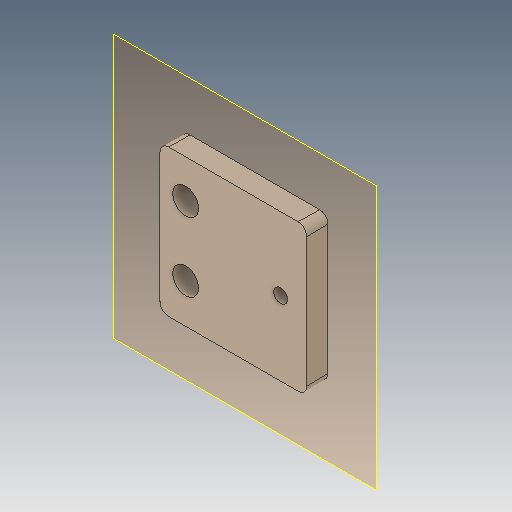
# Autodesk Inventor part: 30_Cube_Z_Focus_Drylin_NEMA_counterplate
Saved by Autodesk Inventor 2019.4 (Build 234330000, 330)
## iProperties
Created: 2021-05-03
Part Number: 30_Cube_Z_Focus_Drylin_NEMA_counterplate
Material: Generic
Document SubType Name: Modeling
Designer: diederichbenedict
Density: 1 g/cm^3
Appearance: Default
Author: diederichbenedict
Autodesk Inventor part; units mm, degrees
ref_plane "YZ Plane" through (0, 0, 0) normal (1, 0, 0) x (0, 1, 0)
ref_plane "XZ Plane" through (0, 0, 0) normal (0, 1, 0) x (-1, 0, 0)
ref_plane "XY Plane" through (0, 0, 0) normal (0, 0, 1) x (1, 0, 0)
ref_plane "Work Plane1" through (15.4052, 15.0652, 4.9) normal (0, 0, 1) x (0, 1, 0)
sketch "Sketch1" plane through (15.4052, 15.0652, 4.9) normal (0, 0, 1) x (0, 1, 0)
  circle A0 centre (5.7948, 15.4052) radius 2.5 projected
  circle A1 centre (-15.6052, -5.7948) radius 2.5 projected
  line L0 (-20.0856, 39.0762) -> (-20.0856, 40.2052) projected
  line L1 (-20.0856, 40.2052) -> (-38.2052, 40.2052) projected
  arc A2 (-38.2052, 40.2052) -> (-40.2052, 38.2052) centre (-38.2052, 38.2052) ccw projected
  line L2 (-40.2052, 20.2953) -> (-40.2052, 38.2052) projected
  line L3 (-40.2052, 20.2953) -> (-39.0783, 20.2953) projected
  arc A3 (-39.0783, 20.2953) -> (-38.6768, 20.6232) centre (-39.0783, 20.7051) ccw projected
  arc A4 (-34.5391, 20.2052) -> (-38.6768, 20.6232) centre (-36.6291, 20.2052) ccw projected
  line L4 (-34.5391, 20.2052) -> (-34.5391, 10.4067) projected
  arc A5 (-38.647, 9.8643) -> (-34.5391, 10.4067) centre (-36.6023, 10.2052) ccw projected
  line L5 (-38.647, 9.8643) -> (-38.6775, 9.9849) projected
  arc A6 (-38.6775, 9.9849) -> (-39.0762, 10.3249) centre (-39.083, 9.9131) ccw projected
  line L6 (-39.0762, 10.3249) -> (-40.2052, 10.3249) projected
  line L7 (-40.2052, -7.7948) -> (-40.2052, 10.3249) projected
  arc A7 (-40.2052, -7.7948) -> (-38.2052, -9.7948) centre (-38.2052, -7.7948) ccw projected
  line L8 (-38.2052, -9.7948) -> (-20.2052, -9.7948) projected
  line L9 (-20.2052, -9.7948) -> (-20.2052, -10.8453) projected
  arc A8 (-20.6052, -11.3352) -> (-20.2052, -10.8453) centre (-20.7052, -10.8453) ccw projected
  arc A9 (-20.6052, -11.3352) -> (-20.2052, -15.2948) centre (-20.2052, -13.2948) ccw projected
  line L10 (-20.2052, -15.2948) -> (-10.2052, -15.2948) projected
  arc A10 (-10.2052, -15.2948) -> (-9.8052, -11.3352) centre (-10.2052, -13.2948) ccw projected
  arc A11 (-10.2052, -10.8453) -> (-9.8052, -11.3352) centre (-9.7052, -10.8453) ccw projected
  line L11 (-10.2052, -10.8453) -> (-10.2052, -9.7948) projected
  line L12 (-10.2052, -9.7948) -> (7.7948, -9.7948) projected
  arc A12 (7.7948, -9.7948) -> (9.7948, -7.7948) centre (7.7948, -7.7948) ccw projected
  line L13 (9.7948, 10.2052) -> (9.7948, -7.7948) projected
  line L14 (9.7948, 10.2052) -> (10.8453, 10.2052) projected
  arc A13 (11.3352, 9.8052) -> (10.8453, 10.2052) centre (10.8453, 9.7052) ccw projected
  arc A14 (11.3352, 9.8052) -> (15.2948, 10.2052) centre (13.2948, 10.2052) ccw projected
  line L15 (15.2948, 10.2052) -> (15.2948, 20.2052) projected
  arc A15 (15.2948, 20.2052) -> (11.3352, 20.6052) centre (13.2948, 20.2052) ccw projected
  arc A16 (10.8453, 20.2052) -> (11.3352, 20.6052) centre (10.8453, 20.7052) ccw projected
  line L16 (10.8453, 20.2052) -> (9.7948, 20.2052) projected
  line L17 (9.7948, 38.2052) -> (9.7948, 20.2052) projected
  arc A17 (9.7948, 38.2052) -> (7.7948, 40.2052) centre (7.7948, 38.2052) ccw projected
  line L18 (7.7948, 40.2052) -> (-10.1151, 40.2052) projected
  line L19 (-10.1151, 40.2052) -> (-10.1151, 39.0783) projected
  arc A18 (-10.1151, 39.0783) -> (-9.7873, 38.6768) centre (-9.7054, 39.0783) ccw projected
  arc A19 (-10.2052, 34.5391) -> (-9.7873, 38.6768) centre (-10.2052, 36.6291) ccw projected
  line L20 (-10.2052, 34.5391) -> (-20.0038, 34.5391) projected
  arc A20 (-20.5462, 38.647) -> (-20.0038, 34.5391) centre (-20.2052, 36.6023) ccw projected
  line L21 (-20.5462, 38.647) -> (-20.4256, 38.6775) projected
  arc A21 (-20.4256, 38.6775) -> (-20.0856, 39.0762) centre (-20.4974, 39.083) ccw projected
  line L22 (-0.2052, 32.2052) -> (-30.2052, 32.2052) projected
  arc A22 (1.7948, 30.2052) -> (-0.2052, 32.2052) centre (-0.2052, 30.2052) ccw projected
  line L23 (1.7948, 30.2052) -> (1.7948, 0.2052) projected
  arc A23 (-0.2052, -1.7948) -> (1.7948, 0.2052) centre (-0.2052, 0.2052) ccw projected
  line L24 (-0.2052, -1.7948) -> (-30.2052, -1.7948) projected
  arc A24 (-32.2052, 0.2052) -> (-30.2052, -1.7948) centre (-30.2052, 0.2052) ccw projected
  line L25 (-32.2052, 0.2052) -> (-32.2052, 30.2052) projected
  arc A25 (-30.2052, 32.2052) -> (-32.2052, 30.2052) centre (-30.2052, 30.2052) ccw projected
  circle A26 centre (-35.2052, 35.2052) radius 2.425 projected
  circle A27 centre (-29.7052, 36.0052) radius 2.65 projected
  circle A28 centre (-36.0052, 29.7052) radius 2.65 projected
  circle A29 centre (-35.2052, -4.7948) radius 2.425 projected
  circle A30 centre (-29.7052, -5.5948) radius 2.65 projected
  circle A31 centre (-36.0052, 0.7052) radius 2.65 projected
  circle A32 centre (4.7948, 35.2052) radius 2.425 projected
  circle A33 centre (-0.7052, 36.0052) radius 2.65 projected
  circle A34 centre (5.5948, 29.7052) radius 2.65 projected
  circle A35 centre (5.5948, 0.7052) radius 2.65 projected
  circle A36 centre (-0.7052, -5.5948) radius 2.65 projected
  circle A37 centre (4.7948, -4.7948) radius 2.425 projected
  point P0 (-15.0652, 15.4052)
extrude "Extrusion1" add sketch "Sketch1" against normal blind 5 draft -1 contours A22 L23 A23 L24 A24 L25 A25 L22
sketch "Sketch2" plane through (15.4052, 15.0652, 4.9) normal (0, 0, 1) x (1, 0, 0)
  circle A0 centre (-26.2552, -7.0652) radius 3 projected
  circle A1 centre (-26.2552, -23.0652) radius 3 projected
  circle A2 centre (-4.2552, -15.0652) radius 1.6 projected
  line L0 (-50.1952, -15.0652) -> (19.3848, -15.0652)
  point P0 (-15.4052, -15.0652)
  constraints: 2 end point, 1 horizontal, 2 other
extrude "Extrusion2" cut sketch "Sketch2" against normal through all
body "Solid1"
